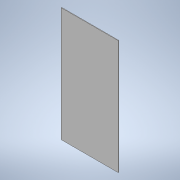
# Autodesk Inventor part: groot plaat
Saved by Autodesk Inventor 2020 (Build 240168000, 168)
## iProperties
Created: 2020-01-14
Part Number: groot plaat
Material: Generic
Document SubType Name: Modeling
Designer: jonas.vandenborne
Density: 1 g/cm^3
Appearance: Default
Author: jonas.vandenborne
Autodesk Inventor part; units mm, degrees
ref_plane "YZ Plane" through (0, 0, 0) normal (1, 0, 0) x (0, 1, 0)
ref_plane "XZ Plane" through (0, 0, 0) normal (0, 1, 0) x (-1, 0, 0)
ref_plane "XY Plane" through (0, 0, 0) normal (0, 0, 1) x (1, 0, 0)
sketch "Sketch1" plane through (0, 0, 0) normal (0, 0, 1) x (1, 0, 0)
  line L0 (0, 0) -> (200, 0)
  line L1 (200, 0) -> (200, 400)
  line L2 (200, 400) -> (0, 400)
  line L3 (0, 400) -> (0, 0)
  dimension "d0" = 200
  dimension "d1" = 400
  constraints: 8 end point, 3 perpendicular, 1 horizontal
  measures "d0" distance of L1.end L2.end
  measures "d1" distance of L0.end L1.end
extrude "Extrusion1" add sketch "Sketch1" against normal blind 2
body "Solid1"
